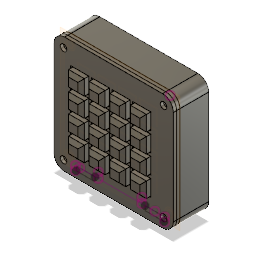
Tastenfeld (Autodesk Fusion 360 design; units mm, degrees)
Autodesk Fusion 360 part; units mm, degrees
note: some values were not read from the file. Chosen so that the rebuilt part matches the saved one: which face or edge a step refers to. Set by a fixed rule: which sketch regions a step uses.
(part 1 of 2)
sketch "Skizze1" plane through (0, 0, 0) normal (0, 0, 1) x (1, 0, 0)
  line L0 (0, 0) -> (39, 0)
  line L1 (39, 0) -> (39, 43.6)
  line L2 (39, 43.6) -> (0, 43.6)
  line L3 (0, 43.6) -> (0, 0)
  dimension "d1" = 39
  dimension "d2" = 43.6
extrude "Extrusion1" add sketch "Skizze1" along normal blind 1.55 makes body 1
sketch "Skizze2" plane through (0, 0, 1.55) normal (0, 0, 1) x (1, 0, 0)
  line L0 (0, 43.6) -> (0, 0)
  line L1 (0, 0) -> (39, 0)
  line L2 (39, 0) -> (39, 43.6)
  line L3 (39, 43.6) -> (0, 43.6)
  line L4 (1, 41.6) -> (6.9, 41.6)
  line L5 (6.9, 41.6) -> (6.9, 35.7)
  line L6 (6.9, 35.7) -> (1, 35.7)
  line L7 (1, 35.7) -> (1, 41.6)
  line L8 (10.5, 35.7) -> (10.5, 41.6)
  line L9 (10.5, 41.6) -> (16.4, 41.6)
  line L10 (16.4, 41.6) -> (16.4, 35.7)
  line L11 (16.4, 35.7) -> (10.5, 35.7)
  line L12 (20, 35.7) -> (20, 41.6)
  line L13 (20, 41.6) -> (25.9, 41.6)
  line L14 (25.9, 41.6) -> (25.9, 35.7)
  line L15 (25.9, 35.7) -> (20, 35.7)
  line L16 (29.5, 35.7) -> (29.5, 41.6)
  line L17 (29.5, 41.6) -> (35.4, 41.6)
  line L18 (35.4, 41.6) -> (35.4, 35.7)
  line L19 (35.4, 35.7) -> (29.5, 35.7)
  line L20 (1, 26.8667) -> (1, 32.7667)
  line L21 (1, 32.7667) -> (6.9, 32.7667)
  line L22 (6.9, 32.7667) -> (6.9, 26.8667)
  line L23 (6.9, 26.8667) -> (1, 26.8667)
  line L24 (10.5, 26.8667) -> (10.5, 32.7667)
  line L25 (10.5, 32.7667) -> (16.4, 32.7667)
  line L26 (16.4, 32.7667) -> (16.4, 26.8667)
  line L27 (16.4, 26.8667) -> (10.5, 26.8667)
  line L28 (20, 26.8667) -> (20, 32.7667)
  line L29 (20, 32.7667) -> (25.9, 32.7667)
  line L30 (25.9, 32.7667) -> (25.9, 26.8667)
  line L31 (25.9, 26.8667) -> (20, 26.8667)
  line L32 (29.5, 26.8667) -> (29.5, 32.7667)
  line L33 (29.5, 32.7667) -> (35.4, 32.7667)
  line L34 (35.4, 32.7667) -> (35.4, 26.8667)
  line L35 (35.4, 26.8667) -> (29.5, 26.8667)
  line L36 (1, 18.0333) -> (1, 23.9333)
  line L37 (1, 23.9333) -> (6.9, 23.9333)
  line L38 (6.9, 23.9333) -> (6.9, 18.0333)
  line L39 (6.9, 18.0333) -> (1, 18.0333)
  line L40 (10.5, 18.0333) -> (10.5, 23.9333)
  line L41 (10.5, 23.9333) -> (16.4, 23.9333)
  line L42 (16.4, 23.9333) -> (16.4, 18.0333)
  line L43 (16.4, 18.0333) -> (10.5, 18.0333)
  line L44 (20, 18.0333) -> (20, 23.9333)
  line L45 (20, 23.9333) -> (25.9, 23.9333)
  line L46 (25.9, 23.9333) -> (25.9, 18.0333)
  line L47 (25.9, 18.0333) -> (20, 18.0333)
  line L48 (29.5, 18.0333) -> (29.5, 23.9333)
  line L49 (29.5, 23.9333) -> (35.4, 23.9333)
  line L50 (35.4, 23.9333) -> (35.4, 18.0333)
  line L51 (35.4, 18.0333) -> (29.5, 18.0333)
  line L52 (1, 9.2) -> (1, 15.1)
  line L53 (1, 15.1) -> (6.9, 15.1)
  line L54 (6.9, 15.1) -> (6.9, 9.2)
  line L55 (6.9, 9.2) -> (1, 9.2)
  line L56 (10.5, 9.2) -> (10.5, 15.1)
  line L57 (10.5, 15.1) -> (16.4, 15.1)
  line L58 (16.4, 15.1) -> (16.4, 9.2)
  line L59 (16.4, 9.2) -> (10.5, 9.2)
  line L60 (20, 9.2) -> (20, 15.1)
  line L61 (20, 15.1) -> (25.9, 15.1)
  line L62 (25.9, 15.1) -> (25.9, 9.2)
  line L63 (25.9, 9.2) -> (20, 9.2)
  line L64 (29.5, 9.2) -> (29.5, 15.1)
  line L65 (29.5, 15.1) -> (35.4, 15.1)
  line L66 (35.4, 15.1) -> (35.4, 9.2)
  line L67 (35.4, 9.2) -> (29.5, 9.2)
  dimension "d5" = 5.9
  dimension "d6" = 5.9
  dimension "d7" = 2
  dimension "d8" = 1
  dimension "d11" = 28.5
  dimension "d12" = -26.5
  measures "d5" distance of L0.end
  measures "d7" distance of L3 L4
  measures "d8" distance of L0 L7
extrude "Extrusion2" add sketch "Skizze2" along normal blind 3.6 contours L4 L5 L6 L7 | L8 L9 L10 L11 | L12 L13 L14 L15 | L16 L17 L18 L19 | L20 L21 L22 L23 | L24 L25 L26 L27 | L28 L29 L30 L31 | L32 L33 L34 L35 | L36 L37 L38 L39 | L40 L41 L42 L43 | L44 L45 L46 L47 | L48 L49 L50 L51 | L52 L53 L54 L55 | L56 L57 L58 L59 | L60 L61 L62 L63 | L64 L65 L66 L67 bodies 1
sketch "Skizze3" plane through (0, 0, 5.15) normal (0, 0, 1) x (1, 0, 0)
  line L0 (1, 35.7) -> (6.9, 35.7)
  line L1 (6.9, 35.7) -> (6.9, 41.6)
  line L2 (6.9, 41.6) -> (1, 41.6)
  line L3 (1, 41.6) -> (1, 35.7)
  circle A0 centre (3.95, 38.65) radius 1.65
  circle A1 centre (13.45, 38.65) radius 1.65
  circle A2 centre (22.95, 38.65) radius 1.65
  circle A3 centre (32.45, 38.65) radius 1.65
  circle A4 centre (3.95, 29.8167) radius 1.65
  circle A5 centre (13.45, 29.8167) radius 1.65
  circle A6 centre (22.95, 29.8167) radius 1.65
  circle A7 centre (32.45, 29.8167) radius 1.65
  circle A8 centre (3.95, 20.9833) radius 1.65
  circle A9 centre (13.45, 20.9833) radius 1.65
  circle A10 centre (22.95, 20.9833) radius 1.65
  circle A11 centre (32.45, 20.9833) radius 1.65
  circle A12 centre (3.95, 12.15) radius 1.65
  circle A13 centre (13.45, 12.15) radius 1.65
  circle A14 centre (22.95, 12.15) radius 1.65
  circle A15 centre (32.45, 12.15) radius 1.65
  dimension "d15" = 3.3
  dimension "d18" = 28.5
  dimension "d19" = -26.5
  measures "d15" diameter of A0
extrude "Extrusion3" add sketch "Skizze3" along normal blind 1.3 contours A0 | A1 | A2 | A3 | A4 | A5 | A6 | A7 | A8 | A9 | A10 | A11 | A12 | A13 | A14 | A15 bodies 1
sketch "Skizze4" plane through (0, 0, 1.55) normal (0, 0, 1) x (1, 0, 0)
  line L0 (6.9, 9.2) -> (1, 9.2)
  line L1 (1, 9.2) -> (1, 15.1)
  line L2 (1, 15.1) -> (6.9, 15.1)
  line L3 (6.9, 15.1) -> (6.9, 9.2)
  line L4 (35.4, 9.2) -> (29.5, 9.2)
  line L5 (29.5, 9.2) -> (29.5, 15.1)
  line L6 (29.5, 15.1) -> (35.4, 15.1)
  line L7 (35.4, 15.1) -> (35.4, 9.2)
  line L8 (6.9, 26.8667) -> (1, 26.8667)
  line L9 (1, 26.8667) -> (1, 32.7667)
  line L10 (1, 32.7667) -> (6.9, 32.7667)
  line L11 (6.9, 32.7667) -> (6.9, 26.8667)
  line L12 (35.4, 35.7) -> (29.5, 35.7)
  line L13 (29.5, 35.7) -> (29.5, 41.6)
  line L14 (29.5, 41.6) -> (35.4, 41.6)
  line L15 (35.4, 41.6) -> (35.4, 35.7)
  line L16 (1, 35.7) -> (1, 41.6)
  line L17 (1, 41.6) -> (6.9, 41.6)
  line L18 (6.9, 41.6) -> (6.9, 35.7)
  line L19 (6.9, 35.7) -> (1, 35.7)
  line L20 (35.4, 26.8667) -> (29.5, 26.8667)
  line L21 (29.5, 26.8667) -> (29.5, 32.7667)
  line L22 (29.5, 32.7667) -> (35.4, 32.7667)
  line L23 (35.4, 32.7667) -> (35.4, 26.8667)
  line L24 (6.9, 18.0333) -> (1, 18.0333)
  line L25 (1, 18.0333) -> (1, 23.9333)
  line L26 (1, 23.9333) -> (6.9, 23.9333)
  line L27 (6.9, 23.9333) -> (6.9, 18.0333)
  line L28 (25.9, 9.2) -> (20, 9.2)
  line L29 (20, 9.2) -> (20, 15.1)
  line L30 (20, 15.1) -> (25.9, 15.1)
  line L31 (25.9, 15.1) -> (25.9, 9.2)
  line L32 (16.4, 9.2) -> (10.5, 9.2)
  line L33 (10.5, 9.2) -> (10.5, 15.1)
  line L34 (10.5, 15.1) -> (16.4, 15.1)
  line L35 (16.4, 15.1) -> (16.4, 9.2)
  line L36 (35.4, 18.0333) -> (29.5, 18.0333)
  line L37 (29.5, 18.0333) -> (29.5, 23.9333)
  line L38 (29.5, 23.9333) -> (35.4, 23.9333)
  line L39 (35.4, 23.9333) -> (35.4, 18.0333)
  line L40 (16.4, 26.8667) -> (10.5, 26.8667)
  line L41 (10.5, 26.8667) -> (10.5, 32.7667)
  line L42 (10.5, 32.7667) -> (16.4, 32.7667)
  line L43 (16.4, 32.7667) -> (16.4, 26.8667)
  line L44 (25.9, 35.7) -> (20, 35.7)
  line L45 (20, 35.7) -> (20, 41.6)
  line L46 (20, 41.6) -> (25.9, 41.6)
  line L47 (25.9, 41.6) -> (25.9, 35.7)
  line L48 (16.4, 35.7) -> (10.5, 35.7)
  line L49 (10.5, 35.7) -> (10.5, 41.6)
  line L50 (10.5, 41.6) -> (16.4, 41.6)
  line L51 (16.4, 41.6) -> (16.4, 35.7)
  line L52 (25.9, 26.8667) -> (20, 26.8667)
  line L53 (20, 26.8667) -> (20, 32.7667)
  line L54 (20, 32.7667) -> (25.9, 32.7667)
  line L55 (25.9, 32.7667) -> (25.9, 26.8667)
  line L56 (16.4, 18.0333) -> (10.5, 18.0333)
  line L57 (10.5, 18.0333) -> (10.5, 23.9333)
  line L58 (10.5, 23.9333) -> (16.4, 23.9333)
  line L59 (16.4, 23.9333) -> (16.4, 18.0333)
  line L60 (25.9, 18.0333) -> (20, 18.0333)
  line L61 (20, 18.0333) -> (20, 23.9333)
  line L62 (20, 23.9333) -> (25.9, 23.9333)
  line L63 (25.9, 23.9333) -> (25.9, 18.0333)
  line L64 (0, 43.6) -> (0, 0)
  line L65 (0, 0) -> (39, 0)
  line L66 (39, 0) -> (39, 43.6)
  line L67 (39, 43.6) -> (0, 43.6)
  line L68 (9.5, 2.6) -> (29.5, 2.6)
  line L69 (29.5, 2.6) -> (29.5, 0.1)
  line L70 (29.5, 0.1) -> (9.5, 0.1)
  line L71 (9.5, 0.1) -> (9.5, 2.6)
  dimension "d22" = 20
  dimension "d23" = 2.5
  dimension "d24" = 9.5
  dimension "d25" = 11
  dimension "d26" = 0.1
  measures "d24" distance of L66 L69
  measures "d25" distance of L64 L71
  measures "d26" distance of L65 L70
extrude "Extrusion4" add sketch "Skizze4" along normal blind 2.5 contours L68 L69 L70 L71 bodies 1
sketch "Skizze5" plane through (0, 0, 4.05) normal (0, 0, 1) x (1, 0, 0)
  line L0 (9.5, 0.1) -> (29.5, 0.1)
  line L1 (29.5, 0.1) -> (29.5, 2.6)
  line L2 (29.5, 2.6) -> (9.5, 2.6)
  line L3 (9.5, 2.6) -> (9.5, 0.1)
  line L4 (10, 1.65) -> (10.6, 1.65)
  line L5 (10.6, 1.65) -> (10.6, 1.05)
  line L6 (10.6, 1.05) -> (10, 1.05)
  line L7 (10, 1.05) -> (10, 1.65)
  line L8 (12.6286, 1.65) -> (13.2286, 1.65)
  line L9 (13.2286, 1.65) -> (13.2286, 1.05)
  line L10 (13.2286, 1.05) -> (12.6286, 1.05)
  line L11 (12.6286, 1.05) -> (12.6286, 1.65)
  line L12 (15.2571, 1.65) -> (15.8571, 1.65)
  line L13 (15.8571, 1.65) -> (15.8571, 1.05)
  line L14 (15.8571, 1.05) -> (15.2571, 1.05)
  line L15 (15.2571, 1.05) -> (15.2571, 1.65)
  line L16 (17.8857, 1.65) -> (18.4857, 1.65)
  line L17 (18.4857, 1.65) -> (18.4857, 1.05)
  line L18 (18.4857, 1.05) -> (17.8857, 1.05)
  line L19 (17.8857, 1.05) -> (17.8857, 1.65)
  line L20 (20.5143, 1.65) -> (21.1143, 1.65)
  line L21 (21.1143, 1.65) -> (21.1143, 1.05)
  line L22 (21.1143, 1.05) -> (20.5143, 1.05)
  line L23 (20.5143, 1.05) -> (20.5143, 1.65)
  line L24 (23.1429, 1.65) -> (23.7429, 1.65)
  line L25 (23.7429, 1.65) -> (23.7429, 1.05)
  line L26 (23.7429, 1.05) -> (23.1429, 1.05)
  line L27 (23.1429, 1.05) -> (23.1429, 1.65)
  line L28 (25.7714, 1.65) -> (26.3714, 1.65)
  line L29 (26.3714, 1.65) -> (26.3714, 1.05)
  line L30 (26.3714, 1.05) -> (25.7714, 1.05)
  line L31 (25.7714, 1.05) -> (25.7714, 1.65)
  line L32 (28.4, 1.65) -> (29, 1.65)
  line L33 (29, 1.65) -> (29, 1.05)
  line L34 (29, 1.05) -> (28.4, 1.05)
  line L35 (28.4, 1.05) -> (28.4, 1.65)
  point P0 (0, -31037849.6)
  dimension "d29" = 0.6
  dimension "d30" = 0.6
  dimension "d31" = 0.5
  dimension "d32" = 0.95
  dimension "d33" = 0.9
  dimension "d34" = 0.5
  dimension "d37" = 18.4
  dimension "d38" = 0
  measures "d31" distance of L3 L7
  measures "d32" distance of L0 L6
  measures "d33" distance of L2 L4
  measures "d34" distance of L1 P0
extrude "Extrusion5" add sketch "Skizze5" along normal blind 0.5 contours L4 L5 L6 L7 | L8 L9 L10 L11 | L12 L13 L14 L15 | L16 L17 L18 L19 | L20 L21 L22 L23 | L24 L25 L26 L27 | L28 L29 L30 L31 | L32 L33 L34 L35 bodies 1
move_face "Flächen versetzen1" offset 6 8 faces at (10.4, 1.05, 4.2167) (13.0286, 1.05, 4.2167) (15.6571, 1.05, 4.2167) (18.2857, 1.05, 4.2167) (20.9143, 1.05, 4.2167) (23.5429, 1.05, 4.2167) (26.1714, 1.05, 4.2167) (28.8, 1.05, 4.2167) on bodies 1
fillet "Abrundung1" radius 0.5 8 edges at (28.7, 1.65, 4.55) (26.0714, 1.65, 4.55) (23.4429, 1.65, 4.55) (20.8143, 1.65, 4.55) (18.1857, 1.65, 4.55) (15.5571, 1.65, 4.55) (12.9286, 1.65, 4.55) (10.3, 1.65, 4.55) on bodies 1
sketch "Skizze6" plane through (0, 0, 0) normal (0, 0, -1) x (-1, 0, 0)
  line L0 (0, 0) -> (0, 43.6)
  line L1 (0, 43.6) -> (-39, 43.6)
  line L2 (-39, 43.6) -> (-39, 0)
  line L3 (-39, 0) -> (0, 0)
  line L4 (-1, 41.6) -> (-35.5, 41.6)
  line L5 (-35.5, 41.6) -> (-35.5, 0)
  line L6 (-35.5, 0) -> (-1, 0)
  line L7 (-1, 0) -> (-1, 41.6)
extrude "Extrusion6" add sketch "Skizze6" along normal blind 1.8 contours L3 L4 L5 L6 L7 bodies 1
sketch "Skizze3 (2)" plane through (0, 0, -1.8) normal (0, 0, -1) x (-1, 0, 0) in component "Component"
  line L0 (-1, 0) -> (-1, 41.6)
  line L1 (-1, 41.6) -> (-35.5, 41.6)
  line L2 (-35.5, 41.6) -> (-35.5, 0)
  line L3 (-35.5, 0) -> (-1, 0)
  line L4 (-47, 51.6) -> (8, 51.6)
  line L5 (8, 51.6) -> (8, -2)
  line L6 (8, -2) -> (-47, -2)
  line L7 (-47, -2) -> (-47, 51.6)
  line L8 (-39, 0) -> (-39, 43.6)
  line L9 (-39, 43.6) -> (0, 43.6)
  line L10 (0, 43.6) -> (0, 0)
  dimension "d260" = 8
  dimension "d261" = 8
  dimension "d262" = 8
  dimension "d263" = 2
  measures "d260" distance of L7 L8
  measures "d261" distance of L4 L9
  measures "d262" distance of L5 L10
  measures "d263" distance of L3 L6
extrude "Extrusion3'" add sketch "Skizze3 (2)" along normal blind 5 separate body contours L0 L1 L2 L3 | L4 L5 L6 L7 makes body 2 in component "Component"
sketch "Skizze4 (2)" plane through (0, 0, -1.8) normal (0, 0, 1) x (1, 0, 0) in component "Component"
  line L0 (-8, -2) -> (47, -2)
  line L1 (47, -2) -> (47, 51.6)
  line L2 (47, 51.6) -> (-8, 51.6)
  line L3 (-8, 51.6) -> (-8, -2)
  circle A0 centre (-3.5, 47.1) radius 1.5
  circle A1 centre (42.5, 47.1) radius 1.5
  circle A2 centre (-3.5, 2.5) radius 1.5
  circle A3 centre (42.5, 2.5) radius 1.5
  dimension "d266" = 3
  dimension "d267" = 4.5
  dimension "d268" = 4.5
  dimension "d269" = 4.5
  dimension "d270" = 4.5
  dimension "d273" = 46
  dimension "d274" = -44.6
  measures "d266" diameter of A0
  measures "d267" distance of L2
  measures "d268" distance of L3
  measures "d269" distance of L1
  measures "d270" distance of L0
extrude "Extrusion4'" cut sketch "Skizze4 (2)" against normal blind 5 contours A0 | A1 | A2 | A3 bodies 2 in component "Component"
sketch "Skizze5 (2)" plane through (0, 0, -6.8) normal (0, 0, -1) x (-1, 0, 0) in component "Component"
  line L0 (-47, -2) -> (8, -2)
  line L1 (8, -2) -> (8, 51.6)
  line L2 (8, 51.6) -> (-47, 51.6)
  line L3 (-47, 51.6) -> (-47, -2)
  line L4 (-44.1166, 49.9) -> (-45.7332, 47.1)
  line L5 (-45.7332, 47.1) -> (-44.1166, 44.3)
  line L6 (-44.1166, 44.3) -> (-40.8834, 44.3)
  line L7 (-40.8834, 44.3) -> (-39.2668, 47.1)
  line L8 (-39.2668, 47.1) -> (-40.8834, 49.9)
  line L9 (-40.8834, 49.9) -> (-44.1166, 49.9)
  line L10 (1.8834, 49.9) -> (0.2668, 47.1)
  line L11 (5.1166, 49.9) -> (1.8834, 49.9)
  line L12 (1.8834, 44.3) -> (5.1166, 44.3)
  circle A0 centre (3.5, 47.1) radius 1.5
  line L13 (6.7332, 47.1) -> (5.1166, 49.9)
  line L14 (0.2668, 47.1) -> (1.8834, 44.3)
  line L15 (5.1166, 44.3) -> (6.7332, 47.1)
  line L16 (-44.1166, 5.3) -> (-45.7332, 2.5)
  line L17 (-40.8834, 5.3) -> (-44.1166, 5.3)
  line L18 (-44.1166, -0.3) -> (-40.8834, -0.3)
  circle A1 centre (-42.5, 2.5) radius 1.5
  line L19 (-39.2668, 2.5) -> (-40.8834, 5.3)
  line L20 (-45.7332, 2.5) -> (-44.1166, -0.3)
  line L21 (-40.8834, -0.3) -> (-39.2668, 2.5)
  line L22 (1.8834, 5.3) -> (0.2668, 2.5)
  line L23 (5.1166, 5.3) -> (1.8834, 5.3)
  line L24 (1.8834, -0.3) -> (5.1166, -0.3)
  circle A2 centre (3.5, 2.5) radius 1.5
  line L25 (6.7332, 2.5) -> (5.1166, 5.3)
  line L26 (0.2668, 2.5) -> (1.8834, -0.3)
  line L27 (5.1166, -0.3) -> (6.7332, 2.5)
  circle A3 centre (-42.5, 47.1) radius 1.5
  circle A4 centre (-42.5, 2.5) radius 1.5
  circle A5 centre (3.5, 47.1) radius 1.5
  circle A6 centre (3.5, 2.5) radius 1.5
  dimension "d277" = 2.8
  dimension "d278" = 4.5
  measures "d278" distance of L2 origin
extrude "Extrusion5'" cut sketch "Skizze5 (2)" against normal blind 2.5 contours L4 L5 L6 L7 L8 L9 | L10 L11 L12 L13 L14 L15 | L16 L17 L18 L19 L20 L21 | L22 L23 L24 L25 L26 L27 bodies 2 in component "Component"
sketch "Skizze6 (2)" plane through (0, 0, -1.8) normal (0, 0, 1) x (1, 0, 0) in component "Component"
  circle A0 centre (42.5, 47.1) radius 1.5
  circle A1 centre (42.5, 2.5) radius 1.5
  circle A2 centre (-3.5, 47.1) radius 1.5
  circle A3 centre (-3.5, 2.5) radius 1.5
  line L0 (-8, -2) -> (47, -2)
  line L1 (47, -2) -> (47, 51.6)
  line L2 (47, 51.6) -> (-8, 51.6)
  line L3 (-8, 51.6) -> (-8, -2)
  line L4 (-6, 0) -> (45, 0)
  line L5 (45, 0) -> (45, 49.6)
  line L6 (45, 49.6) -> (-6, 49.6)
  line L7 (-6, 49.6) -> (-6, 0)
  circle A4 centre (-3.5, 47.1) radius 2.5
  circle A5 centre (42.5, 47.1) radius 2.5
  circle A6 centre (42.5, 2.5) radius 2.5
  circle A7 centre (-3.5, 2.5) radius 2.5
  dimension "d285" = 2
  measures "d285" distance of L0
extrude "Extrusion6'" add sketch "Skizze6 (2)" along normal blind 8.3 contours L0 L1 L2 L3 | L4 L7 A7 | A7 | L4 L5 A6 | A6 | L6 L7 A4 | A4 | L5 L6 A5 bodies 2 in component "Component"
sketch "Skizze7" plane through (0, -2, 0) normal (0, -1, 0) x (1, 0, 0) in component "Component"
  line L0 (-8, 6.5) -> (-8, -6.8)
  line L1 (-8, -6.8) -> (47, -6.8)
  line L2 (47, -6.8) -> (47, 6.5)
  line L3 (47, 6.5) -> (-8, 6.5)
  line L4 (-1, 6.5) -> (40, 6.5)
  line L5 (40, 6.5) -> (40, -1.8)
  line L6 (40, -1.8) -> (-1, -1.8)
  line L7 (-1, -1.8) -> (-1, 6.5)
  line L8 (29, 4.05) -> (29, 4.55)
  line L9 (29, 4.05) -> (28.4, 4.05)
  dimension "d295" = 7
  dimension "d296" = 7
  dimension "d297" = 5
  measures "d295" distance of L2 L5
  measures "d296" distance of L0 L7
  measures "d297" distance of L1 L6
extrude "Extrusion7" cut sketch "Skizze7" against normal blind 2 contours L3 L4 L5 L6 L7 bodies 2 in component "Component"
sketch "Skizze8" plane through (0, 0, 6.5) normal (0, 0, 1) x (1, 0, 0) in component "Component"
  circle A0 centre (-3.5, 2.5) radius 1.5
  line L0 (-1, -2) -> (-1, 0)
  line L1 (-1, 0) -> (-3.5, 0)
  arc A1 (-3.5, 0) -> (-6, 2.5) centre (-3.5, 2.5) ccw
  line L2 (-6, 2.5) -> (-6, 47.1)
  arc A2 (-6, 47.1) -> (-3.5, 49.6) centre (-3.5, 47.1) ccw
  line L3 (-3.5, 49.6) -> (42.5, 49.6)
  arc A3 (45, 47.1) -> (42.5, 49.6) centre (42.5, 47.1) ccw
  line L4 (45, 47.1) -> (45, 2.5)
  arc A4 (45, 2.5) -> (42.5, 0) centre (42.5, 2.5) ccw
  line L5 (42.5, 0) -> (40, 0)
  line L6 (40, 0) -> (40, -2)
  line L7 (40, -2) -> (47, -2)
  line L8 (47, -2) -> (47, 51.6)
  line L9 (47, 51.6) -> (-8, 51.6)
  line L10 (-8, 51.6) -> (-8, -2)
  line L11 (-8, -2) -> (-1, -2)
  circle A5 centre (-3.5, 47.1) radius 1.5
  circle A6 centre (42.5, 2.5) radius 1.5
sketch "Skizze9" plane through (0, 0, -1.8) normal (0, 0, 1) x (1, 0, 0) in component "Component"
  line L0 (0, 0) -> (-1, 0)
  line L1 (-1, 0) -> (-1, 45)
  line L2 (-1, 45) -> (0, 45)
  line L3 (0, 45) -> (0, 0)
  line L4 (40, 0) -> (35.8, 0)
  line L5 (35.8, 0) -> (35.8, 45)
  line L6 (35.8, 45) -> (40, 45)
  line L7 (40, 45) -> (40, 0)
  line L8 (0, 0) -> (0.7, 0)
  line L9 (0.7, 0) -> (0.7, 45)
  line L10 (0.7, 45) -> (0, 45)
  line L11 (0, 45) -> (0, 0)
  line L12 (35.5, 0) -> (35.5, 41.6)
  line L13 (0.7, 45) -> (35.8, 45)
  line L14 (35.8, 45) -> (35.8, 41.9)
  line L15 (35.8, 41.9) -> (0.7, 41.9)
  line L16 (0.7, 41.9) -> (0.7, 45)
  line L17 (1, 41.6) -> (35.5, 41.6)
  dimension "d298" = 45
  dimension "d299" = 1
  dimension "d301" = 0.3
  dimension "d302" = 0.3
  dimension "d305" = 0.3
  measures "d301" distance of L5 L12
  measures "d302" distance of L15 L17
extrude "Extrusion9" add sketch "Skizze9" along normal blind 1.5 separate body makes body 3 in component "Component"
extrude "Extrusion10" add sketch "Skizze6 (2)" along normal blind 8.3 contours A5 bodies 2 in component "Component"
fillet "Abrundung1'" radius 5 4 edges at (47, -2, -0.15) (47, 51.6, -0.15) (-8, 51.6, -0.15) (-8, -2, -0.15) on bodies 2 in component "Component"
sketch "Skizze1 (2)" plane through (0, 0, 6.5) normal (0, 0, 1) x (1, 0, 0) in component "Component'"
  line L0 (-8, 51.6) -> (47, 51.6)
  line L1 (47, 51.6) -> (47, -2)
  line L2 (47, -2) -> (-8, -2)
  line L3 (-8, -2) -> (-8, 51.6)
  circle A0 centre (-3.5, 47.1) radius 1.5
  circle A1 centre (42.5, 47.1) radius 1.5
  circle A2 centre (42.5, 2.5) radius 1.5
  circle A3 centre (-3.5, 2.5) radius 1.5
  line L4 (0.3, 34.1) -> (-0.2, 34.1)
  line L5 (-0.2, 34.1) -> (-0.2, 41.4)
  line L6 (-0.2, 41.4) -> (0.3, 41.4)
  line L7 (0.3, 41.4) -> (0.3, 34.1)
  line L8 (7.6, 34.1) -> (8.1, 34.1)
  line L9 (8.1, 34.1) -> (8.1, 41.6)
  line L10 (8.1, 41.6) -> (7.6, 41.6)
  line L11 (7.6, 41.6) -> (7.6, 34.1)
  line L12 (7.6, 41.6) -> (-0.2, 41.6)
  line L13 (-0.2, 41.6) -> (-0.2, 41.1)
  line L14 (-0.2, 41.1) -> (7.6, 41.1)
  line L15 (7.6, 41.1) -> (7.6, 41.6)
  line L16 (9.8, 34.1) -> (9.3, 34.1)
  line L17 (17.1, 41.6) -> (17.1, 34.1)
  line L18 (17.1, 41.1) -> (17.1, 41.6)
  line L19 (9.8, 41.4) -> (9.8, 34.1)
  line L20 (17.1, 34.1) -> (17.6, 34.1)
  line L21 (9.3, 34.1) -> (9.3, 41.4)
  line L22 (17.1, 41.6) -> (9.3, 41.6)
  line L23 (9.3, 41.6) -> (9.3, 41.1)
  line L24 (9.3, 41.1) -> (17.1, 41.1)
  line L25 (17.6, 41.6) -> (17.1, 41.6)
  line L26 (17.6, 34.1) -> (17.6, 41.6)
  line L27 (9.3, 41.4) -> (9.8, 41.4)
  line L28 (19.3, 34.1) -> (18.8, 34.1)
  line L29 (26.6, 41.6) -> (26.6, 34.1)
  line L30 (26.6, 41.1) -> (26.6, 41.6)
  line L31 (19.3, 41.4) -> (19.3, 34.1)
  line L32 (26.6, 34.1) -> (27.1, 34.1)
  line L33 (18.8, 34.1) -> (18.8, 41.4)
  line L34 (26.6, 41.6) -> (18.8, 41.6)
  line L35 (18.8, 41.6) -> (18.8, 41.1)
  line L36 (18.8, 41.1) -> (26.6, 41.1)
  line L37 (27.1, 41.6) -> (26.6, 41.6)
  line L38 (27.1, 34.1) -> (27.1, 41.6)
  line L39 (18.8, 41.4) -> (19.3, 41.4)
  line L40 (28.8, 34.1) -> (28.3, 34.1)
  line L41 (36.1, 41.6) -> (36.1, 34.1)
  line L42 (36.1, 41.1) -> (36.1, 41.6)
  line L43 (28.8, 41.4) -> (28.8, 34.1)
  line L44 (36.1, 34.1) -> (36.6, 34.1)
  line L45 (28.3, 34.1) -> (28.3, 41.4)
  line L46 (36.1, 41.6) -> (28.3, 41.6)
  line L47 (28.3, 41.6) -> (28.3, 41.1)
  line L48 (28.3, 41.1) -> (36.1, 41.1)
  line L49 (36.6, 41.6) -> (36.1, 41.6)
  line L50 (36.6, 34.1) -> (36.6, 41.6)
  line L51 (28.3, 41.4) -> (28.8, 41.4)
  line L52 (0.3, 25.2667) -> (-0.2, 25.2667)
  line L53 (7.6, 32.7667) -> (7.6, 25.2667)
  line L54 (7.6, 32.2667) -> (7.6, 32.7667)
  line L55 (0.3, 32.5667) -> (0.3, 25.2667)
  line L56 (7.6, 25.2667) -> (8.1, 25.2667)
  line L57 (-0.2, 25.2667) -> (-0.2, 32.5667)
  line L58 (7.6, 32.7667) -> (-0.2, 32.7667)
  line L59 (-0.2, 32.7667) -> (-0.2, 32.2667)
  line L60 (-0.2, 32.2667) -> (7.6, 32.2667)
  line L61 (8.1, 32.7667) -> (7.6, 32.7667)
  line L62 (8.1, 25.2667) -> (8.1, 32.7667)
  line L63 (-0.2, 32.5667) -> (0.3, 32.5667)
  line L64 (9.8, 25.2667) -> (9.3, 25.2667)
  line L65 (17.1, 32.7667) -> (17.1, 25.2667)
  line L66 (17.1, 32.2667) -> (17.1, 32.7667)
  line L67 (9.8, 32.5667) -> (9.8, 25.2667)
  line L68 (17.1, 25.2667) -> (17.6, 25.2667)
  line L69 (9.3, 25.2667) -> (9.3, 32.5667)
  line L70 (17.1, 32.7667) -> (9.3, 32.7667)
  line L71 (9.3, 32.7667) -> (9.3, 32.2667)
  line L72 (9.3, 32.2667) -> (17.1, 32.2667)
  line L73 (17.6, 32.7667) -> (17.1, 32.7667)
  line L74 (17.6, 25.2667) -> (17.6, 32.7667)
  line L75 (9.3, 32.5667) -> (9.8, 32.5667)
  line L76 (19.3, 25.2667) -> (18.8, 25.2667)
  line L77 (26.6, 32.7667) -> (26.6, 25.2667)
  line L78 (26.6, 32.2667) -> (26.6, 32.7667)
  line L79 (19.3, 32.5667) -> (19.3, 25.2667)
  line L80 (26.6, 25.2667) -> (27.1, 25.2667)
  line L81 (18.8, 25.2667) -> (18.8, 32.5667)
  line L82 (26.6, 32.7667) -> (18.8, 32.7667)
  line L83 (18.8, 32.7667) -> (18.8, 32.2667)
  line L84 (18.8, 32.2667) -> (26.6, 32.2667)
  line L85 (27.1, 32.7667) -> (26.6, 32.7667)
  line L86 (27.1, 25.2667) -> (27.1, 32.7667)
  line L87 (18.8, 32.5667) -> (19.3, 32.5667)
  line L88 (28.8, 25.2667) -> (28.3, 25.2667)
  line L89 (36.1, 32.7667) -> (36.1, 25.2667)
  line L90 (36.1, 32.2667) -> (36.1, 32.7667)
  line L91 (28.8, 32.5667) -> (28.8, 25.2667)
  line L92 (36.1, 25.2667) -> (36.6, 25.2667)
  line L93 (28.3, 25.2667) -> (28.3, 32.5667)
  line L94 (36.1, 32.7667) -> (28.3, 32.7667)
  line L95 (28.3, 32.7667) -> (28.3, 32.2667)
  line L96 (28.3, 32.2667) -> (36.1, 32.2667)
  line L97 (36.6, 32.7667) -> (36.1, 32.7667)
  line L98 (36.6, 25.2667) -> (36.6, 32.7667)
  line L99 (28.3, 32.5667) -> (28.8, 32.5667)
  line L100 (0.3, 16.4333) -> (-0.2, 16.4333)
  line L101 (7.6, 23.9333) -> (7.6, 16.4333)
  line L102 (7.6, 23.4333) -> (7.6, 23.9333)
  line L103 (0.3, 23.7333) -> (0.3, 16.4333)
  line L104 (7.6, 16.4333) -> (8.1, 16.4333)
  line L105 (-0.2, 16.4333) -> (-0.2, 23.7333)
  line L106 (7.6, 23.9333) -> (-0.2, 23.9333)
  line L107 (-0.2, 23.9333) -> (-0.2, 23.4333)
  line L108 (-0.2, 23.4333) -> (7.6, 23.4333)
  line L109 (8.1, 23.9333) -> (7.6, 23.9333)
  line L110 (8.1, 16.4333) -> (8.1, 23.9333)
  line L111 (-0.2, 23.7333) -> (0.3, 23.7333)
  line L112 (9.8, 16.4333) -> (9.3, 16.4333)
  line L113 (17.1, 23.9333) -> (17.1, 16.4333)
  line L114 (17.1, 23.4333) -> (17.1, 23.9333)
  line L115 (9.8, 23.7333) -> (9.8, 16.4333)
  line L116 (17.1, 16.4333) -> (17.6, 16.4333)
  line L117 (9.3, 16.4333) -> (9.3, 23.7333)
  line L118 (17.1, 23.9333) -> (9.3, 23.9333)
  line L119 (9.3, 23.9333) -> (9.3, 23.4333)
  line L120 (9.3, 23.4333) -> (17.1, 23.4333)
  line L121 (17.6, 23.9333) -> (17.1, 23.9333)
  line L122 (17.6, 16.4333) -> (17.6, 23.9333)
  line L123 (9.3, 23.7333) -> (9.8, 23.7333)
  line L124 (19.3, 16.4333) -> (18.8, 16.4333)
  line L125 (26.6, 23.9333) -> (26.6, 16.4333)
  line L126 (26.6, 23.4333) -> (26.6, 23.9333)
  line L127 (19.3, 23.7333) -> (19.3, 16.4333)
  line L128 (26.6, 16.4333) -> (27.1, 16.4333)
  line L129 (18.8, 16.4333) -> (18.8, 23.7333)
  line L130 (26.6, 23.9333) -> (18.8, 23.9333)
  line L131 (18.8, 23.9333) -> (18.8, 23.4333)
  line L132 (18.8, 23.4333) -> (26.6, 23.4333)
  line L133 (27.1, 23.9333) -> (26.6, 23.9333)
  line L134 (27.1, 16.4333) -> (27.1, 23.9333)
  line L135 (18.8, 23.7333) -> (19.3, 23.7333)
  line L136 (28.8, 16.4333) -> (28.3, 16.4333)
  line L137 (36.1, 23.9333) -> (36.1, 16.4333)
  line L138 (36.1, 23.4333) -> (36.1, 23.9333)
  line L139 (28.8, 23.7333) -> (28.8, 16.4333)
  line L140 (36.1, 16.4333) -> (36.6, 16.4333)
  line L141 (28.3, 16.4333) -> (28.3, 23.7333)
  line L142 (36.1, 23.9333) -> (28.3, 23.9333)
  line L143 (28.3, 23.9333) -> (28.3, 23.4333)
  line L144 (28.3, 23.4333) -> (36.1, 23.4333)
  line L145 (36.6, 23.9333) -> (36.1, 23.9333)
  line L146 (36.6, 16.4333) -> (36.6, 23.9333)
  line L147 (28.3, 23.7333) -> (28.8, 23.7333)
  line L148 (0.3, 7.6) -> (-0.2, 7.6)
  line L149 (7.6, 15.1) -> (7.6, 7.6)
  line L150 (7.6, 14.6) -> (7.6, 15.1)
  line L151 (0.3, 14.9) -> (0.3, 7.6)
  line L152 (7.6, 7.6) -> (8.1, 7.6)
  line L153 (-0.2, 7.6) -> (-0.2, 14.9)
  line L154 (7.6, 15.1) -> (-0.2, 15.1)
  line L155 (-0.2, 15.1) -> (-0.2, 14.6)
  line L156 (-0.2, 14.6) -> (7.6, 14.6)
  line L157 (8.1, 15.1) -> (7.6, 15.1)
  line L158 (8.1, 7.6) -> (8.1, 15.1)
  line L159 (-0.2, 14.9) -> (0.3, 14.9)
  line L160 (9.8, 7.6) -> (9.3, 7.6)
  line L161 (17.1, 15.1) -> (17.1, 7.6)
  line L162 (17.1, 14.6) -> (17.1, 15.1)
  line L163 (9.8, 14.9) -> (9.8, 7.6)
  line L164 (17.1, 7.6) -> (17.6, 7.6)
  line L165 (9.3, 7.6) -> (9.3, 14.9)
  line L166 (17.1, 15.1) -> (9.3, 15.1)
  line L167 (9.3, 15.1) -> (9.3, 14.6)
  line L168 (9.3, 14.6) -> (17.1, 14.6)
  line L169 (17.6, 15.1) -> (17.1, 15.1)
  line L170 (17.6, 7.6) -> (17.6, 15.1)
  line L171 (9.3, 14.9) -> (9.8, 14.9)
  line L172 (19.3, 7.6) -> (18.8, 7.6)
  line L173 (26.6, 15.1) -> (26.6, 7.6)
  line L174 (26.6, 14.6) -> (26.6, 15.1)
  line L175 (19.3, 14.9) -> (19.3, 7.6)
  line L176 (26.6, 7.6) -> (27.1, 7.6)
  line L177 (18.8, 7.6) -> (18.8, 14.9)
  line L178 (26.6, 15.1) -> (18.8, 15.1)
  line L179 (18.8, 15.1) -> (18.8, 14.6)
  line L180 (18.8, 14.6) -> (26.6, 14.6)
  line L181 (27.1, 15.1) -> (26.6, 15.1)
  line L182 (27.1, 7.6) -> (27.1, 15.1)
  line L183 (18.8, 14.9) -> (19.3, 14.9)
  line L184 (28.8, 7.6) -> (28.3, 7.6)
  line L185 (36.1, 15.1) -> (36.1, 7.6)
  line L186 (36.1, 14.6) -> (36.1, 15.1)
  line L187 (28.8, 14.9) -> (28.8, 7.6)
  line L188 (36.1, 7.6) -> (36.6, 7.6)
  line L189 (28.3, 7.6) -> (28.3, 14.9)
  line L190 (36.1, 15.1) -> (28.3, 15.1)
  line L191 (28.3, 15.1) -> (28.3, 14.6)
  line L192 (28.3, 14.6) -> (36.1, 14.6)
  line L193 (36.6, 15.1) -> (36.1, 15.1)
  line L194 (36.6, 7.6) -> (36.6, 15.1)
  line L195 (28.3, 14.9) -> (28.8, 14.9)
  line L196 (-1, 45) -> (-1, 0)
  dimension "d309" = 0.5
  dimension "d312" = 28.5
  dimension "d313" = -26.5
  dimension "d323" = 7.3
  dimension "d324" = 7
  dimension "d325" = 7
  dimension "d327" = 0.5
  dimension "d328" = 0.8
  dimension "d329" = 10
  measures "d323" distance of L7 L11
  measures "d324" distance of L14
  measures "d325" distance of origin L14
  measures "d327" distance of L12 L14
  measures "d328" distance of L5 L196
  measures "d329" distance of L0 L12
extrude "Extrusion1'" add sketch "Skizze1 (2)" along normal blind 1.5 separate body makes body 4 in component "Component'"
fillet "Abrundung1''" radius 5 4 edges at (47, -2, 7.25) (47, 51.6, 7.25) (-8, 51.6, 7.25) (-8, -2, 7.25) on bodies 4 in component "Component'"
sketch "Skizze2 (2)" plane through (0, 0, 6.5) normal (0, 0, -1) x (-1, 0, 0) in component "Component'"
  line L0 (-0.3, 32.2667) -> (-7.6, 32.2667)
  line L1 (-7.6, 32.2667) -> (-7.6, 25.2667)
  line L2 (-7.6, 25.2667) -> (-8.1, 25.2667)
  line L3 (-8.1, 25.2667) -> (-8.1, 32.7667)
  line L4 (-8.1, 32.7667) -> (0.2, 32.7667)
  line L5 (0.2, 32.7667) -> (0.2, 25.2667)
  line L6 (0.2, 25.2667) -> (-0.3, 25.2667)
  line L7 (-0.3, 25.2667) -> (-0.3, 32.2667)
  line L8 (-9.8, 23.4333) -> (-17.1, 23.4333)
  line L9 (-17.1, 23.4333) -> (-17.1, 16.4333)
  line L10 (-17.1, 16.4333) -> (-17.6, 16.4333)
  line L11 (-17.6, 16.4333) -> (-17.6, 23.9333)
  line L12 (-17.6, 23.9333) -> (-9.3, 23.9333)
  line L13 (-9.3, 23.9333) -> (-9.3, 16.4333)
  line L14 (-9.3, 16.4333) -> (-9.8, 16.4333)
  line L15 (-9.8, 16.4333) -> (-9.8, 23.4333)
  line L16 (-19.3, 23.4333) -> (-26.6, 23.4333)
  line L17 (-26.6, 23.4333) -> (-26.6, 16.4333)
  line L18 (-26.6, 16.4333) -> (-27.1, 16.4333)
  line L19 (-27.1, 16.4333) -> (-27.1, 23.9333)
  line L20 (-27.1, 23.9333) -> (-18.8, 23.9333)
  line L21 (-18.8, 23.9333) -> (-18.8, 16.4333)
  line L22 (-18.8, 16.4333) -> (-19.3, 16.4333)
  line L23 (-19.3, 16.4333) -> (-19.3, 23.4333)
  line L24 (-28.8, 23.4333) -> (-36.1, 23.4333)
  line L25 (-36.1, 23.4333) -> (-36.1, 16.4333)
  line L26 (-36.1, 16.4333) -> (-36.6, 16.4333)
  line L27 (-36.6, 16.4333) -> (-36.6, 23.9333)
  line L28 (-36.6, 23.9333) -> (-28.3, 23.9333)
  line L29 (-28.3, 23.9333) -> (-28.3, 16.4333)
  line L30 (-28.3, 16.4333) -> (-28.8, 16.4333)
  line L31 (-28.8, 16.4333) -> (-28.8, 23.4333)
  line L32 (-0.3, 14.6) -> (-7.6, 14.6)
  line L33 (-7.6, 14.6) -> (-7.6, 7.6)
  line L34 (-7.6, 7.6) -> (-8.1, 7.6)
  line L35 (-8.1, 7.6) -> (-8.1, 15.1)
  line L36 (-8.1, 15.1) -> (0.2, 15.1)
  line L37 (0.2, 15.1) -> (0.2, 7.6)
  line L38 (0.2, 7.6) -> (-0.3, 7.6)
  line L39 (-0.3, 7.6) -> (-0.3, 14.6)
  line L40 (-0.3, 23.4333) -> (-7.6, 23.4333)
  line L41 (-7.6, 23.4333) -> (-7.6, 16.4333)
  line L42 (-7.6, 16.4333) -> (-8.1, 16.4333)
  line L43 (-8.1, 16.4333) -> (-8.1, 23.9333)
  line L44 (-8.1, 23.9333) -> (0.2, 23.9333)
  line L45 (0.2, 23.9333) -> (0.2, 16.4333)
  line L46 (0.2, 16.4333) -> (-0.3, 16.4333)
  line L47 (-0.3, 16.4333) -> (-0.3, 23.4333)
  line L48 (-28.8, 32.2667) -> (-36.1, 32.2667)
  line L49 (-36.1, 32.2667) -> (-36.1, 25.2667)
  line L50 (-36.1, 25.2667) -> (-36.6, 25.2667)
  line L51 (-36.6, 25.2667) -> (-36.6, 32.7667)
  line L52 (-36.6, 32.7667) -> (-28.3, 32.7667)
  line L53 (-28.3, 32.7667) -> (-28.3, 25.2667)
  line L54 (-28.3, 25.2667) -> (-28.8, 25.2667)
  line L55 (-28.8, 25.2667) -> (-28.8, 32.2667)
  line L56 (-19.3, 32.2667) -> (-26.6, 32.2667)
  line L57 (-26.6, 32.2667) -> (-26.6, 25.2667)
  line L58 (-26.6, 25.2667) -> (-27.1, 25.2667)
  line L59 (-27.1, 25.2667) -> (-27.1, 32.7667)
  line L60 (-27.1, 32.7667) -> (-18.8, 32.7667)
  line L61 (-18.8, 32.7667) -> (-18.8, 25.2667)
  line L62 (-18.8, 25.2667) -> (-19.3, 25.2667)
  line L63 (-19.3, 25.2667) -> (-19.3, 32.2667)
  line L64 (-9.8, 32.2667) -> (-17.1, 32.2667)
  line L65 (-17.1, 32.2667) -> (-17.1, 25.2667)
  line L66 (-17.1, 25.2667) -> (-17.6, 25.2667)
  line L67 (-17.6, 25.2667) -> (-17.6, 32.7667)
  line L68 (-17.6, 32.7667) -> (-9.3, 32.7667)
  line L69 (-9.3, 32.7667) -> (-9.3, 25.2667)
  line L70 (-9.3, 25.2667) -> (-9.8, 25.2667)
  line L71 (-9.8, 25.2667) -> (-9.8, 32.2667)
  line L72 (-28.8, 41.1) -> (-36.1, 41.1)
  line L73 (-36.1, 41.1) -> (-36.1, 34.1)
  line L74 (-36.1, 34.1) -> (-36.6, 34.1)
  line L75 (-36.6, 34.1) -> (-36.6, 41.6)
  line L76 (-36.6, 41.6) -> (-28.3, 41.6)
  line L77 (-28.3, 41.6) -> (-28.3, 34.1)
  line L78 (-28.3, 34.1) -> (-28.8, 34.1)
  line L79 (-28.8, 34.1) -> (-28.8, 41.1)
  line L80 (-19.3, 41.1) -> (-26.6, 41.1)
  line L81 (-26.6, 41.1) -> (-26.6, 34.1)
  line L82 (-26.6, 34.1) -> (-27.1, 34.1)
  line L83 (-27.1, 34.1) -> (-27.1, 41.6)
  line L84 (-27.1, 41.6) -> (-18.8, 41.6)
  line L85 (-18.8, 41.6) -> (-18.8, 34.1)
  line L86 (-18.8, 34.1) -> (-19.3, 34.1)
  line L87 (-19.3, 34.1) -> (-19.3, 41.1)
  circle A0 centre (3.5, 2.5) radius 1.5
  line L88 (-9.8, 41.1) -> (-17.1, 41.1)
  line L89 (-17.1, 41.1) -> (-17.1, 34.1)
  line L90 (-17.1, 34.1) -> (-17.6, 34.1)
  line L91 (-17.6, 34.1) -> (-17.6, 41.6)
  line L92 (-17.6, 41.6) -> (-9.3, 41.6)
  line L93 (-9.3, 41.6) -> (-9.3, 34.1)
  line L94 (-9.3, 34.1) -> (-9.8, 34.1)
  line L95 (-9.8, 34.1) -> (-9.8, 41.1)
  circle A1 centre (-42.5, 2.5) radius 1.5
  circle A2 centre (-42.5, 47.1) radius 1.5
  circle A3 centre (3.5, 47.1) radius 1.5
  line L96 (-0.3, 41.1) -> (-7.6, 41.1)
  line L97 (-7.6, 41.1) -> (-7.6, 34.1)
  line L98 (-7.6, 34.1) -> (-8.1, 34.1)
  line L99 (-8.1, 34.1) -> (-8.1, 41.6)
  line L100 (-8.1, 41.6) -> (0.2, 41.6)
  line L101 (0.2, 41.6) -> (0.2, 34.1)
  line L102 (0.2, 34.1) -> (-0.3, 34.1)
  line L103 (-0.3, 34.1) -> (-0.3, 41.1)
  line L104 (-9.8, 14.6) -> (-17.1, 14.6)
  line L105 (-17.1, 14.6) -> (-17.1, 7.6)
  line L106 (-17.1, 7.6) -> (-17.6, 7.6)
  line L107 (-17.6, 7.6) -> (-17.6, 15.1)
  line L108 (-17.6, 15.1) -> (-9.3, 15.1)
  line L109 (-9.3, 15.1) -> (-9.3, 7.6)
  line L110 (-9.3, 7.6) -> (-9.8, 7.6)
  line L111 (-9.8, 7.6) -> (-9.8, 14.6)
  line L112 (-19.3, 14.6) -> (-26.6, 14.6)
  line L113 (-26.6, 14.6) -> (-26.6, 7.6)
  line L114 (-26.6, 7.6) -> (-27.1, 7.6)
  line L115 (-27.1, 7.6) -> (-27.1, 15.1)
  line L116 (-27.1, 15.1) -> (-18.8, 15.1)
  line L117 (-18.8, 15.1) -> (-18.8, 7.6)
  line L118 (-18.8, 7.6) -> (-19.3, 7.6)
  line L119 (-19.3, 7.6) -> (-19.3, 14.6)
  line L120 (-28.8, 14.6) -> (-36.1, 14.6)
  line L121 (-36.1, 14.6) -> (-36.1, 7.6)
  line L122 (-36.1, 7.6) -> (-36.6, 7.6)
  line L123 (-36.6, 7.6) -> (-36.6, 15.1)
  line L124 (-36.6, 15.1) -> (-28.3, 15.1)
  line L125 (-28.3, 15.1) -> (-28.3, 7.6)
  line L126 (-28.3, 7.6) -> (-28.8, 7.6)
  line L127 (-28.8, 7.6) -> (-28.8, 14.6)
  arc A4 (3, -2) -> (8, 3) centre (3, 3) ccw
  line L128 (8, 3) -> (8, 46.6)
  arc A5 (8, 46.6) -> (3, 51.6) centre (3, 46.6) ccw
  line L129 (3, 51.6) -> (-42, 51.6)
  arc A6 (-42, 51.6) -> (-47, 46.6) centre (-42, 46.6) ccw
  line L130 (-47, 46.6) -> (-47, 3)
  arc A7 (-47, 3) -> (-42, -2) centre (-42, 3) ccw
  line L131 (-42, -2) -> (3, -2)
  line L132 (-40, 45) -> (-37.1, 45)
  line L133 (-37.1, 45) -> (-37.1, 6)
  line L134 (-37.1, 6) -> (-40, 6)
  line L135 (-40, 6) -> (-40, 45)
  line L136 (-37.1, 45) -> (1, 45)
  line L137 (1, 45) -> (1, 42.1)
  line L138 (1, 42.1) -> (-37.1, 42.1)
  line L139 (-37.1, 42.1) -> (-37.1, 45)
  line L140 (1, 45) -> (1, 0)
  line L141 (1, 42.1) -> (0.7, 42.1)
  line L142 (0.7, 42.1) -> (0.7, 6)
  line L143 (0.7, 6) -> (1, 6)
  line L144 (1, 6) -> (1, 42.1)
  line L145 (1, 8) -> (-40, 8)
  line L146 (-40, 8) -> (-40, 6)
  line L147 (-40, 6) -> (1, 6)
  line L148 (1, 6) -> (1, 8)
  line L149 (-16.6, 8.5) -> (-10.3, 8.5)
  dimension "d317" = 0.5
  dimension "d318" = 0.5
  dimension "d319" = 0.5
  dimension "d320" = 0.5
  measures "d317" distance of L123 L133
  measures "d318" distance of L76 L138
  measures "d319" distance of L37 L142
  measures "d320" distance of L145 L149
sketch "Skizze10" plane through (0, 0, -0.3) normal (0, 0, 1) x (1, 0, 0) in component "Component"
  line L0 (40, 45) -> (-1, 45)
  line L1 (-1, 45) -> (-1, 0)
  line L2 (-1, 0) -> (0.7, 0)
  line L3 (0.7, 0) -> (0.7, 41.9)
  line L4 (0.7, 41.9) -> (35.8, 41.9)
  line L5 (35.8, 41.9) -> (35.8, 0)
  line L6 (35.8, 0) -> (40, 0)
  line L7 (40, 0) -> (40, 45)
  line L8 (-1, 45) -> (40, 45)
  line L9 (40, 45) -> (40, 43.61)
  line L10 (40, 43.61) -> (-1, 43.61)
  line L11 (-1, 43.61) -> (-1, 45)
  line L12 (39, 43.6) -> (0, 43.6)
  line L13 (40, 0) -> (39.3, 0)
  line L14 (39.3, 0) -> (39.3, 43.61)
  line L15 (39.3, 43.61) -> (40, 43.61)
  line L16 (40, 43.61) -> (40, 0)
  line L17 (39, 0) -> (39, 43.6)
  line L18 (-1, 43.61) -> (-0.3, 43.61)
  line L19 (-0.3, 43.61) -> (-0.3, 0)
  line L20 (-0.3, 0) -> (-1, 0)
  line L21 (-1, 0) -> (-1, 43.61)
  line L22 (0, 43.6) -> (0, 0)
  dimension "d330" = 0.01
  dimension "d331" = 0.3
  dimension "d332" = 0.3
  measures "d330" distance of L10 L12
  measures "d331" distance of L14 L17
  measures "d332" distance of L19 L22
extrude "Extrusion11" add sketch "Skizze10" along normal blind 2.1 contours L0 L1 L7 L8 L9 L10 L11 L15 L18 | L6 L7 L10 L13 L14 L15 L16 | L1 L2 L10 L18 L19 L20 L21 bodies 3 2 in component "Component"
sketch "Skizze3 (3)" plane through (0, 0, 6.5) normal (0, 0, -1) x (-1, 0, 0) in component "Component'"
  circle A0 centre (-42.5, 2.5) radius 1.5
  line L0 (-36.1, 34.1) -> (-36.6, 34.1)
  line L1 (-36.6, 34.1) -> (-36.6, 41.6)
  line L2 (-36.6, 41.6) -> (-28.3, 41.6)
  line L3 (-28.3, 41.6) -> (-28.3, 34.1)
  line L4 (-28.3, 34.1) -> (-28.8, 34.1)
  line L5 (-28.8, 34.1) -> (-28.8, 41.1)
  line L6 (-28.8, 41.1) -> (-36.1, 41.1)
  line L7 (-36.1, 41.1) -> (-36.1, 34.1)
  line L8 (-26.6, 34.1) -> (-27.1, 34.1)
  line L9 (-27.1, 34.1) -> (-27.1, 41.6)
  line L10 (-27.1, 41.6) -> (-18.8, 41.6)
  line L11 (-18.8, 41.6) -> (-18.8, 34.1)
  line L12 (-18.8, 34.1) -> (-19.3, 34.1)
  line L13 (-19.3, 34.1) -> (-19.3, 41.1)
  line L14 (-19.3, 41.1) -> (-26.6, 41.1)
  line L15 (-26.6, 41.1) -> (-26.6, 34.1)
  line L16 (-17.1, 34.1) -> (-17.6, 34.1)
  line L17 (-17.6, 34.1) -> (-17.6, 41.6)
  line L18 (-17.6, 41.6) -> (-9.3, 41.6)
  line L19 (-9.3, 41.6) -> (-9.3, 34.1)
  line L20 (-9.3, 34.1) -> (-9.8, 34.1)
  line L21 (-9.8, 34.1) -> (-9.8, 41.1)
  line L22 (-9.8, 41.1) -> (-17.1, 41.1)
  line L23 (-17.1, 41.1) -> (-17.1, 34.1)
  circle A1 centre (3.5, 2.5) radius 1.5
  circle A2 centre (-42.5, 47.1) radius 1.5
  circle A3 centre (3.5, 47.1) radius 1.5
  line L24 (-17.1, 7.6) -> (-17.6, 7.6)
  line L25 (-17.6, 7.6) -> (-17.6, 15.1)
  line L26 (-17.6, 15.1) -> (-9.3, 15.1)
  line L27 (-9.3, 15.1) -> (-9.3, 7.6)
  line L28 (-9.3, 7.6) -> (-9.8, 7.6)
  line L29 (-9.8, 7.6) -> (-9.8, 14.6)
  line L30 (-9.8, 14.6) -> (-17.1, 14.6)
  line L31 (-17.1, 14.6) -> (-17.1, 7.6)
  line L32 (-26.6, 7.6) -> (-27.1, 7.6)
  line L33 (-27.1, 7.6) -> (-27.1, 15.1)
  line L34 (-27.1, 15.1) -> (-18.8, 15.1)
  line L35 (-18.8, 15.1) -> (-18.8, 7.6)
  line L36 (-18.8, 7.6) -> (-19.3, 7.6)
  line L37 (-19.3, 7.6) -> (-19.3, 14.6)
  line L38 (-19.3, 14.6) -> (-26.6, 14.6)
  line L39 (-26.6, 14.6) -> (-26.6, 7.6)
  line L40 (-17.1, 25.2667) -> (-17.6, 25.2667)
  line L41 (-17.6, 25.2667) -> (-17.6, 32.7667)
  line L42 (-17.6, 32.7667) -> (-9.3, 32.7667)
  line L43 (-9.3, 32.7667) -> (-9.3, 25.2667)
  line L44 (-9.3, 25.2667) -> (-9.8, 25.2667)
  line L45 (-9.8, 25.2667) -> (-9.8, 32.2667)
  line L46 (-9.8, 32.2667) -> (-17.1, 32.2667)
  line L47 (-17.1, 32.2667) -> (-17.1, 25.2667)
  line L48 (-36.1, 7.6) -> (-36.6, 7.6)
  line L49 (-36.6, 7.6) -> (-36.6, 15.1)
  line L50 (-36.6, 15.1) -> (-28.3, 15.1)
  line L51 (-28.3, 15.1) -> (-28.3, 7.6)
  line L52 (-28.3, 7.6) -> (-28.8, 7.6)
  line L53 (-28.8, 7.6) -> (-28.8, 14.6)
  line L54 (-28.8, 14.6) -> (-36.1, 14.6)
  line L55 (-36.1, 14.6) -> (-36.1, 7.6)
  line L56 (-8.1, 41.6) -> (0.2, 41.6)
  line L57 (0.2, 41.6) -> (0.2, 34.1)
  line L58 (0.2, 34.1) -> (-0.3, 34.1)
  line L59 (-0.3, 34.1) -> (-0.3, 41.1)
  line L60 (-0.3, 41.1) -> (-7.6, 41.1)
  line L61 (-7.6, 41.1) -> (-7.6, 34.1)
  line L62 (-7.6, 34.1) -> (-8.1, 34.1)
  line L63 (-8.1, 34.1) -> (-8.1, 41.6)
  line L64 (-7.6, 25.2667) -> (-8.1, 25.2667)
  line L65 (-8.1, 25.2667) -> (-8.1, 32.7667)
  line L66 (-8.1, 32.7667) -> (0.2, 32.7667)
  line L67 (0.2, 32.7667) -> (0.2, 25.2667)
  line L68 (0.2, 25.2667) -> (-0.3, 25.2667)
  line L69 (-0.3, 25.2667) -> (-0.3, 32.2667)
  line L70 (-0.3, 32.2667) -> (-7.6, 32.2667)
  line L71 (-7.6, 32.2667) -> (-7.6, 25.2667)
  line L72 (-7.6, 16.4333) -> (-8.1, 16.4333)
  line L73 (-8.1, 16.4333) -> (-8.1, 23.9333)
  line L74 (-8.1, 23.9333) -> (0.2, 23.9333)
  line L75 (0.2, 23.9333) -> (0.2, 16.4333)
  line L76 (0.2, 16.4333) -> (-0.3, 16.4333)
  line L77 (-0.3, 16.4333) -> (-0.3, 23.4333)
  line L78 (-0.3, 23.4333) -> (-7.6, 23.4333)
  line L79 (-7.6, 23.4333) -> (-7.6, 16.4333)
  line L80 (-7.6, 7.6) -> (-8.1, 7.6)
  line L81 (-8.1, 7.6) -> (-8.1, 15.1)
  line L82 (-8.1, 15.1) -> (0.2, 15.1)
  line L83 (0.2, 15.1) -> (0.2, 7.6)
  line L84 (0.2, 7.6) -> (-0.3, 7.6)
  line L85 (-0.3, 7.6) -> (-0.3, 14.6)
  line L86 (-0.3, 14.6) -> (-7.6, 14.6)
  line L87 (-7.6, 14.6) -> (-7.6, 7.6)
  line L88 (-36.1, 16.4333) -> (-36.6, 16.4333)
  line L89 (-36.6, 16.4333) -> (-36.6, 23.9333)
  line L90 (-36.6, 23.9333) -> (-28.3, 23.9333)
  line L91 (-28.3, 23.9333) -> (-28.3, 16.4333)
  line L92 (-28.3, 16.4333) -> (-28.8, 16.4333)
  line L93 (-28.8, 16.4333) -> (-28.8, 23.4333)
  line L94 (-28.8, 23.4333) -> (-36.1, 23.4333)
  line L95 (-36.1, 23.4333) -> (-36.1, 16.4333)
  line L96 (-26.6, 16.4333) -> (-27.1, 16.4333)
  line L97 (-27.1, 16.4333) -> (-27.1, 23.9333)
  line L98 (-27.1, 23.9333) -> (-18.8, 23.9333)
  line L99 (-18.8, 23.9333) -> (-18.8, 16.4333)
  line L100 (-18.8, 16.4333) -> (-19.3, 16.4333)
  line L101 (-19.3, 16.4333) -> (-19.3, 23.4333)
  line L102 (-19.3, 23.4333) -> (-26.6, 23.4333)
  line L103 (-26.6, 23.4333) -> (-26.6, 16.4333)
  line L104 (-17.1, 16.4333) -> (-17.6, 16.4333)
  line L105 (-17.6, 16.4333) -> (-17.6, 23.9333)
  line L106 (-17.6, 23.9333) -> (-9.3, 23.9333)
  line L107 (-9.3, 23.9333) -> (-9.3, 16.4333)
  line L108 (-9.3, 16.4333) -> (-9.8, 16.4333)
  line L109 (-9.8, 16.4333) -> (-9.8, 23.4333)
  line L110 (-9.8, 23.4333) -> (-17.1, 23.4333)
  line L111 (-17.1, 23.4333) -> (-17.1, 16.4333)
  line L112 (-36.1, 25.2667) -> (-36.6, 25.2667)
  line L113 (-36.6, 25.2667) -> (-36.6, 32.7667)
  line L114 (-36.6, 32.7667) -> (-28.3, 32.7667)
  line L115 (-28.3, 32.7667) -> (-28.3, 25.2667)
  line L116 (-28.3, 25.2667) -> (-28.8, 25.2667)
  line L117 (-28.8, 25.2667) -> (-28.8, 32.2667)
  line L118 (-28.8, 32.2667) -> (-36.1, 32.2667)
  line L119 (-36.1, 32.2667) -> (-36.1, 25.2667)
  line L120 (-26.6, 25.2667) -> (-27.1, 25.2667)
  line L121 (-27.1, 25.2667) -> (-27.1, 32.7667)
  line L122 (-27.1, 32.7667) -> (-18.8, 32.7667)
  line L123 (-18.8, 32.7667) -> (-18.8, 25.2667)
  line L124 (-18.8, 25.2667) -> (-19.3, 25.2667)
  line L125 (-19.3, 25.2667) -> (-19.3, 32.2667)
  line L126 (-19.3, 32.2667) -> (-26.6, 32.2667)
  line L127 (-26.6, 32.2667) -> (-26.6, 25.2667)
  arc A4 (3, -2) -> (8, 3) centre (3, 3) ccw
  line L128 (8, 3) -> (8, 46.6)
  arc A5 (8, 46.6) -> (3, 51.6) centre (3, 46.6) ccw
  line L129 (3, 51.6) -> (-42, 51.6)
  arc A6 (-42, 51.6) -> (-47, 46.6) centre (-42, 46.6) ccw
  line L130 (-47, 46.6) -> (-47, 3)
  arc A7 (-47, 3) -> (-42, -2) centre (-42, 3) ccw
  line L131 (-42, -2) -> (3, -2)
  line L132 (0.7, -2) -> (-8, -2)
  line L133 (-8, -2) -> (-8, 0)
  line L134 (-8, 0) -> (0.7, 0)
  line L135 (0.7, 0) -> (0.7, -2)
  line L136 (-35.5, 0) -> (-1, 0)
  line L137 (-39.7, -2) -> (-31, -2)
  line L138 (-31, -2) -> (-31, 0)
  line L139 (-31, 0) -> (-39.7, 0)
  line L140 (-39.7, 0) -> (-39.7, -2)
  line L141 (-40, 0) -> (-40, -2)
  line L142 (1, -2) -> (1, 0)
  line L143 (-9.5, 0.1) -> (-9.5, 2.6)
  line L144 (-29.5, 2.6) -> (-29.5, 0.1)
  dimension "d335" = 0.3
  dimension "d336" = 0.3
  dimension "d337" = 1.5
  dimension "d338" = 1.5
  measures "d335" distance of L140 L141
  measures "d336" distance of L135 L142
  measures "d337" distance of L133 L143
  measures "d338" distance of L138 L144
extrude "Extrusion3''" add sketch "Skizze3 (3)" along normal blind 8 contours L131 L132 L133 L134 L135 L136 | L131 L136 L137 L138 L139 L140 bodies 4 in component "Component'"